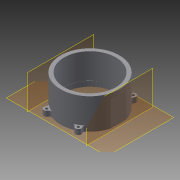
# Autodesk Inventor part: feed_pipe
Saved by Autodesk Inventor 2014 SP2 (Build 180246200, 246)
## iProperties
Created: 2015-11-29
Part Number: feed_pipe
Material: Generic
Document SubType Name: Modeling
Designer: schrluka
Density: 1 g/cm^3
Appearance: Default
Author: schrluka
Autodesk Inventor part; units mm, degrees
ref_plane "YZ Plane" through (0, 0, 0) normal (1, 0, 0) x (0, 1, 0)
ref_plane "XZ Plane" through (0, 0, 0) normal (0, 1, 0) x (-1, 0, 0)
ref_plane "XY Plane" through (0, 0, 0) normal (0, 0, 1) x (1, 0, 0)
ref_plane "Work Plane1" through (0, 0, 0) normal (0, 0, 1) x (1, 0, 0)
sketch "Sketch1" plane through (0, 0, 0) normal (0, 0, 1) x (1, 0, 0)
  arc A0 (31.171, 56.4627) -> (24.1706, 58.6976) centre (26.6395, 54.3496) ccw projected
  arc A1 (24.1706, 58.6976) -> (23.3311, 58.2129) centre (57.5, 0) ccw projected
  arc A2 (23.3311, 58.2129) -> (21.7664, 51.0329) centre (25.8621, 53.9008) ccw projected
  arc A3 (20.857, 44.3118) -> (21.7664, 51.0329) centre (17.6706, 48.165) ccw projected
  arc A4 (20.857, 44.3118) -> (3.8552, 20.7) centre (57.5, 0) ccw projected
  arc A5 (-0.8095, 17.5) -> (3.8552, 20.7) centre (-0.8095, 22.5) ccw projected
  line L0 (-0.8095, 17.5) -> (-27, 17.5) projected
  arc A6 (-27, 17.5) -> (-32, 12.5) centre (-27, 12.5) ccw projected
  line L1 (-32, -12.5) -> (-32, 12.5) projected
  arc A7 (-32, -12.5) -> (-27, -17.5) centre (-27, -12.5) ccw projected
  line L2 (-0.8095, -17.5) -> (-27, -17.5) projected
  arc A8 (3.8552, -20.7) -> (-0.8095, -17.5) centre (-0.8095, -22.5) ccw projected
  arc A9 (3.8552, -20.7) -> (20.857, -44.3118) centre (57.5, 0) ccw projected
  arc A10 (21.7664, -51.0329) -> (20.857, -44.3118) centre (17.6706, -48.165) ccw projected
  arc A11 (21.7664, -51.0329) -> (23.3311, -58.2129) centre (25.8621, -53.9008) ccw projected
  arc A12 (23.3311, -58.2129) -> (24.1706, -58.6976) centre (57.5, 0) ccw projected
  arc A13 (24.1706, -58.6976) -> (31.171, -56.4627) centre (26.6395, -54.3496) ccw projected
  arc A14 (37.4464, -53.8897) -> (31.171, -56.4627) centre (35.7026, -58.5758) ccw projected
  arc A15 (37.4464, -53.8897) -> (77.5536, -53.8897) centre (57.5, 0) ccw projected
  arc A16 (83.829, -56.4627) -> (77.5536, -53.8897) centre (79.2974, -58.5758) ccw projected
  arc A17 (83.829, -56.4627) -> (90.8294, -58.6976) centre (88.3605, -54.3496) ccw projected
  arc A18 (90.8294, -58.6976) -> (91.6689, -58.2129) centre (57.5, 0) ccw projected
  arc A19 (91.6689, -58.2129) -> (93.2336, -51.0329) centre (89.1379, -53.9008) ccw projected
  arc A20 (94.143, -44.3118) -> (93.2336, -51.0329) centre (97.3294, -48.165) ccw projected
  arc A21 (94.143, -44.3118) -> (111.1448, -20.7) centre (57.5, 0) ccw projected
  arc A22 (115.8095, -17.5) -> (111.1448, -20.7) centre (115.8095, -22.5) ccw projected
  line L3 (115.8095, -17.5) -> (142, -17.5) projected
  arc A23 (142, -17.5) -> (147, -12.5) centre (142, -12.5) ccw projected
  line L4 (147, -12.5) -> (147, 12.5) projected
  arc A24 (147, 12.5) -> (142, 17.5) centre (142, 12.5) ccw projected
  line L5 (115.8095, 17.5) -> (142, 17.5) projected
  arc A25 (111.1448, 20.7) -> (115.8095, 17.5) centre (115.8095, 22.5) ccw projected
  arc A26 (111.1448, 20.7) -> (94.143, 44.3118) centre (57.5, 0) ccw projected
  arc A27 (93.2336, 51.0329) -> (94.143, 44.3118) centre (97.3294, 48.165) ccw projected
  arc A28 (93.2336, 51.0329) -> (91.6689, 58.2129) centre (89.1379, 53.9008) ccw projected
  arc A29 (91.6689, 58.2129) -> (90.8294, 58.6976) centre (57.5, 0) ccw projected
  arc A30 (90.8294, 58.6976) -> (83.829, 56.4627) centre (88.3605, 54.3496) ccw projected
  arc A31 (77.5536, 53.8897) -> (83.829, 56.4627) centre (79.2974, 58.5758) ccw projected
  arc A32 (77.5536, 53.8897) -> (37.4464, 53.8897) centre (57.5, 0) ccw projected
  arc A33 (31.171, 56.4627) -> (37.4464, 53.8897) centre (35.7026, 58.5758) ccw projected
  circle A34 centre (26.4765, 53.7343) radius 2.5 projected
  circle A35 centre (88.5235, 53.7343) radius 2.5 projected
  circle A36 centre (26.4765, -53.7343) radius 2.5 projected
  circle A37 centre (88.5235, -53.7343) radius 2.5 projected
  arc A38 (107.5799, -6.5) -> (108, 0) centre (57.5, 0) ccw projected
  line L6 (55.9485, 15.6873) -> (38.0892, 46.6205) projected
  arc A39 (53.812, 4.7327) -> (55.9485, 15.6873) centre (48.5872, 11.4373) ccw projected
  arc A40 (53.812, 4.7327) -> (51.5573, 0.8276) centre (57.5, 0) ccw projected
  arc A41 (43.1386, -6.5) -> (51.5573, 0.8276) centre (43.1386, 2) ccw projected
  line L7 (7.4201, -6.5) -> (43.1386, -6.5) projected
  arc A42 (82.75, 43.7343) -> (76.9108, 46.6205) centre (57.5, 0) ccw projected
  line L8 (44.6901, -9.1873) -> (26.8309, -40.1205) projected
  arc A43 (55.2454, -5.5603) -> (44.6901, -9.1873) centre (52.0513, -13.4373) ccw projected
  arc A44 (55.2454, -5.5603) -> (59.7546, -5.5603) centre (57.5, 0) ccw projected
  arc A45 (70.3099, -9.1873) -> (59.7546, -5.5603) centre (62.9487, -13.4373) ccw projected
  line L9 (88.1691, -40.1205) -> (70.3099, -9.1873) projected
  circle A46 centre (57.5, 0) radius 4.5 projected
  arc A47 (38.0892, 46.6205) -> (32.25, 43.7343) centre (57.5, 0) ccw projected
  line L10 (71.8614, -6.5) -> (107.5799, -6.5) projected
  arc A48 (63.4427, 0.8276) -> (71.8614, -6.5) centre (71.8614, 2) ccw projected
  arc A49 (63.4427, 0.8276) -> (61.188, 4.7327) centre (57.5, 0) ccw projected
  arc A50 (59.0515, 15.6873) -> (61.188, 4.7327) centre (66.4128, 11.4373) ccw projected
  line L11 (76.9108, 46.6205) -> (59.0515, 15.6873) projected
  arc A51 (-1.0279, -13) -> (-1.0279, -10) centre (-1.0279, -11.5) ccw projected
  line L12 (-1.0279, -13) -> (-4.0279, -13) projected
  arc A52 (-4.0279, -10) -> (-4.0279, -13) centre (-4.0279, -11.5) ccw projected
  line L13 (-4.0279, -10) -> (-1.0279, -10) projected
  arc A53 (-27.0279, 13) -> (-27.0279, 10) centre (-27.0279, 11.5) ccw projected
  line L14 (-27.0279, 13) -> (-24.0279, 13) projected
  arc A54 (-24.0279, 10) -> (-24.0279, 13) centre (-24.0279, 11.5) ccw projected
  line L15 (-24.0279, 10) -> (-27.0279, 10) projected
  arc A55 (-27.0279, -10) -> (-27.0279, -13) centre (-27.0279, -11.5) ccw projected
  line L16 (-27.0279, -10) -> (-24.0279, -10) projected
  arc A56 (-24.0279, -13) -> (-24.0279, -10) centre (-24.0279, -11.5) ccw projected
  line L17 (-24.0279, -13) -> (-27.0279, -13) projected
  arc A57 (-4.0279, 13) -> (-4.0279, 10) centre (-4.0279, 11.5) ccw projected
  line L18 (-4.0279, 13) -> (-1.0279, 13) projected
  arc A58 (-1.0279, 10) -> (-1.0279, 13) centre (-1.0279, 11.5) ccw projected
  line L19 (-1.0279, 10) -> (-4.0279, 10) projected
  circle A59 centre (-14.0279, 0) radius 12 projected
  line L20 (139.0279, -10) -> (142.0279, -10) projected
  arc A60 (142.0279, -13) -> (142.0279, -10) centre (142.0279, -11.5) ccw projected
  line L21 (142.0279, -13) -> (139.0279, -13) projected
  arc A61 (139.0279, -10) -> (139.0279, -13) centre (139.0279, -11.5) ccw projected
  arc A62 (139.0279, 13) -> (139.0279, 10) centre (139.0279, 11.5) ccw projected
  line L22 (139.0279, 13) -> (142.0279, 13) projected
  arc A63 (142.0279, 10) -> (142.0279, 13) centre (142.0279, 11.5) ccw projected
  line L23 (142.0279, 10) -> (139.0279, 10) projected
  line L24 (119.0279, -13) -> (116.0279, -13) projected
  arc A64 (116.0279, -10) -> (116.0279, -13) centre (116.0279, -11.5) ccw projected
  line L25 (116.0279, -10) -> (119.0279, -10) projected
  arc A65 (119.0279, -13) -> (119.0279, -10) centre (119.0279, -11.5) ccw projected
  arc A66 (116.0279, 13) -> (116.0279, 10) centre (116.0279, 11.5) ccw projected
  line L26 (116.0279, 13) -> (119.0279, 13) projected
  arc A67 (119.0279, 10) -> (119.0279, 13) centre (119.0279, 11.5) ccw projected
  line L27 (119.0279, 10) -> (116.0279, 10) projected
  circle A68 centre (129.0279, 0) radius 12 projected
  arc A69 (3.8552, 20.7) -> (3.8552, -20.7) centre (57.5, 0) ccw
  arc A70 (110.415, -22.5) -> (111.1448, 20.7) centre (57.5, 0) ccw
  arc A71 (76.9108, 46.6205) -> (38.0892, 46.6205) centre (57.5, 0) ccw
  arc A72 (7.4201, -6.5) -> (26.8309, -40.1205) centre (57.5, 0) ccw
  arc A73 (88.1691, -40.1205) -> (107.5799, -6.5) centre (57.5, 0) ccw
  arc A74 (82.75, -43.7343) -> (88.1691, -40.1205) centre (57.5, 0) ccw projected
  line L28 (82.75, -43.7343) -> (82.6429, -43.5487) projected
  line L29 (32.3571, -43.5487) -> (32.25, -43.7343) projected
  arc A75 (107.7857, 0) -> (82.6429, 43.5487) centre (57.5, 0) ccw projected
  line L30 (107.7857, 0) -> (108, 0) projected
  line L31 (82.75, 43.7343) -> (82.6429, 43.5487) projected
  arc A76 (32.3571, 43.5487) -> (7.2143, 0) centre (57.5, 0) ccw projected
  line L32 (32.3571, 43.5487) -> (32.25, 43.7343) projected
  arc A77 (7, 0) -> (7.4201, -6.5) centre (57.5, 0) ccw projected
  line L33 (7, 0) -> (7.2143, 0) projected
  arc A78 (32.3571, -43.5487) -> (82.6429, -43.5487) centre (57.5, 0) ccw projected
  arc A79 (26.8309, -40.1205) -> (32.25, -43.7343) centre (57.5, 0) ccw projected
  point P0 (0, 0)
  constraints: 11 point on circle, 5 centre point, 5 coincident
extrude "Extrusion1" add sketch "Sketch1" along normal blind 10 contours A33 A32 A31 A30 A29 A28 A27 A26 A70 A21 A20 A19 A18 A17 A16 A15 A14 A13 A12 A11 A10 A9 A69 A4 A3 A2 A1 A0
sketch "Sketch2" plane through (0, 0, 10) normal (0, 0, 1) x (1, 0, 0)
  circle A0 centre (57.5, 0) radius 50.5 projected
  circle A1 centre (57.5, 0) radius 57.5
  point P0 (0, 0)
  constraints: 1 centre point, 1 coincident
extrude "Extrusion2" add sketch "Sketch2" along normal blind 50
ref_plane "Work Plane3" through (0, 0, 0) normal (1, 0, 0) x (0, 1, 0)
ref_plane "Work Plane2" through (0.0721, 14.1, 45) normal (1, 0, 0) x (0, -1, 0)
sketch "Sketch3" plane through (0, 0, 0) normal (1, 0, 0) x (0, 1, 0)
  line L0 (17.533, 50) -> (-17.533, 50)
  line L1 (-17.533, 50) -> (-17.533, 0)
  line L2 (-17.533, 0) -> (17.533, 0)
  line L3 (17.533, 0) -> (17.533, 50)
  line L4 (17.533, 50) -> (-17.533, 0) construction
  line L5 (-17.533, 50) -> (17.533, 0) construction
  point P0 (0, 0)
  point P1 (0, 25)
  dimension "d4" = 50
  constraints: 12 end point, 2 midpoint, 2 parallel, 1 horizontal, 1 perpendicular
  measures "d4" distance of L0.end L1.end
extrude "Extrusion3" cut sketch "Sketch3" along normal blind 2
ref_plane "Work Plane6" through (115, 0, 0) normal (1, 0, 0) x (0, 1, 0)
ref_plane "Work Plane5" through (147, 0, -2.5) normal (1, 0, 0) x (0, -1, 0)
sketch "Sketch4" plane through (115, 0, 0) normal (1, 0, 0) x (0, 1, 0)
  line L0 (15.0333, 0) -> (15.0333, 50) projected
  line L1 (-15.0333, 50) -> (-15.0333, 0) projected
  line L2 (15.0333, 50) -> (-15.0333, 50) projected
  line L3 (15.0333, 0) -> (15.0333, 50) projected
  line L4 (-15.0333, 0) -> (15.0333, 0) projected
  point P0 (0, 0)
extrude "Extrusion4" cut sketch "Sketch4" against normal blind 2
body "Solid1"
